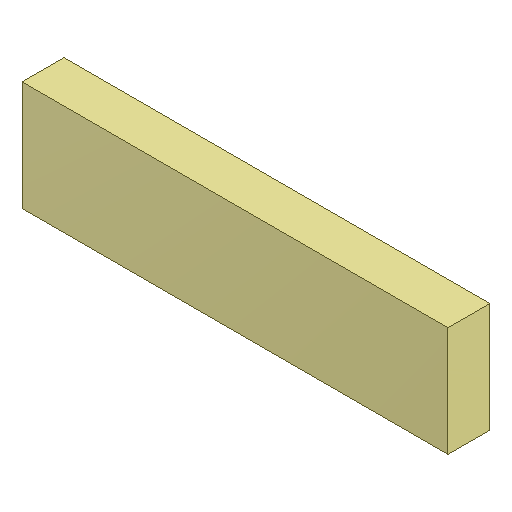
# Autodesk Inventor part: MA04-1
Saved by Autodesk Inventor 2022 (Build 260153000, 153)
## iProperties
Created: 2022-01-18
Part Number: MA04-1
Material: Generisch
Document SubType Name: Modeling
Designer: diederichbenedict
Density: 1 g/cm^3
Appearance: MA04-1, MA04-1
Author: diederichbenedict
Autodesk Inventor part; units mm, degrees
ref_plane "YZ Plane" through (0, 0, 0) normal (1, 0, 0) x (0, 1, 0)
ref_plane "XZ Plane" through (0, 0, 0) normal (0, 1, 0) x (-1, 0, 0)
ref_plane "XY Plane" through (0, 0, 0) normal (0, 0, 1) x (1, 0, 0)
sketch "MA04-1, MA04-1_9" plane through (0, 0, 0) normal (0, 0, 1) x (1, 0, 0)
  line L0 (-5.08, 1.3462) -> (5.08, 1.3462)
  line L1 (5.08, 1.3462) -> (5.08, -1.27)
  line L2 (5.08, -1.27) -> (-5.08, -1.27)
  line L3 (-5.08, -1.27) -> (-5.08, 1.3462)
  constraints: 8 end point
extrude "Extrusion1" add sketch "MA04-1, MA04-1_9" along normal blind 1
